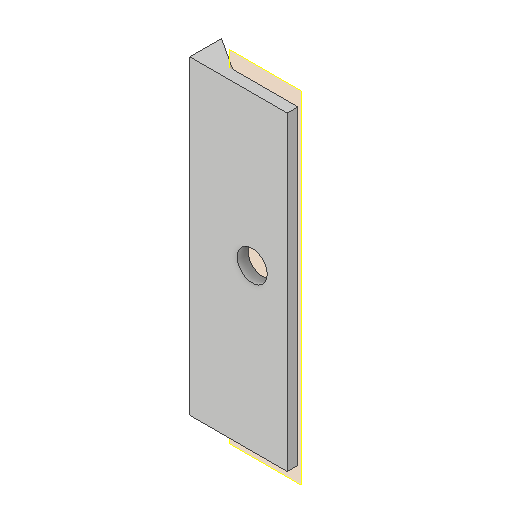
# Autodesk Inventor part: cellSTORM_v5_chiptry_clamp
Saved by Autodesk Inventor 2022 (Build 260153000, 153)
## iProperties
Created: 2020-05-10
Part Number: cellSTORM_v5_chiptry_clamp
Material: Generic
Document SubType Name: Modeling
Designer: diederichbenedict
Density: 1 g/cm^3
Appearance: Default
Author: diederichbenedict
Autodesk Inventor part; units mm, degrees
ref_plane "YZ Plane" through (0, 0, 0) normal (1, 0, 0) x (0, 1, 0)
ref_plane "XZ Plane" through (0, 0, 0) normal (0, 1, 0) x (-1, 0, 0)
ref_plane "XY Plane" through (0, 0, 0) normal (0, 0, 1) x (1, 0, 0)
ref_plane "Work Plane1" through (0, 0, 0) normal (0, 0, 1) x (1, 0, 0)
sketch "Sketch1" plane through (0, 0, 0) normal (0, 0, 1) x (1, 0, 0)
  arc A0 (0, 9.6831) -> (0, 20.3535) centre (0, 15.0183) ccw projected
  line L0 (0, 0) -> (0, 9.6831) projected
  line L1 (6.1022, 0) -> (0, 0) projected
  line L2 (6.1022, 0) -> (6.1022, 29) projected
  line L3 (6.1022, 29) -> (0, 29) projected
  line L4 (0, 20.3535) -> (0, 29) projected
  line L5 (6.1022, 29) -> (-3, 29)
  line L6 (-3, 29) -> (-3, 0)
  line L7 (-3, 0) -> (6.1022, 0)
  line L8 (6.1022, 0) -> (6.1022, 29)
  circle A1 centre (2.8309, 15.0183) radius 1.4 projected
  dimension "d0" = 3
  constraints: 8 end point, 2 parallel, 1 horizontal, 1 perpendicular
  measures "d0" distance between parallel lines of L6 L0
extrude "Extrusion1" add sketch "Sketch1" along normal blind 1
sketch "Sketch2" plane through (-3, 0, 0) normal (0, -1, 0) x (1, 0, 0)
  line L0 (0, 0) -> (9.1022, 0) projected
  line L1 (9.1022, 0) -> (9.1022, 1) projected
  line L2 (0, 1) -> (9.1022, 1) projected
  line L3 (0, 0) -> (0, 1) projected
  line L4 (-3.1221, -0.6) -> (3.4779, -0.6)
  line L5 (9.1022, 0) -> (0, 0) projected
  line L6 (0, 0) -> (3, 0)
  line L7 (0, 0) -> (0, -1.9574)
  line L8 (0, -1.9574) -> (3, 0)
  point P0 (0, -0.6)
  constraints: 8 end point, 1 collinear, 1 horizontal, 1 point on line, 1 vertical, 2 other
extrude "Extrusion2" add sketch "Sketch2" against normal up to surface (29 mm away) contours L0 L8 L4 L7 | L4 L8 L7
body "Solid1"
